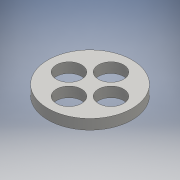
# Autodesk Inventor part: wheel
Saved by Autodesk Inventor 2016 (Build 200138000, 138)
## iProperties
Created: 2016-04-07
Part Number: wheel
Material: Generic
Document SubType Name: Modeling
Designer: hesaon
Density: 1 g/cm^3
Appearance: Default
Author: hesaon
Autodesk Inventor part; units mm, degrees
ref_plane "YZ Plane" through (0, 0, 0) normal (1, 0, 0) x (0, 1, 0)
ref_plane "XZ Plane" through (0, 0, 0) normal (0, 1, 0) x (-1, 0, 0)
ref_plane "XY Plane" through (0, 0, 0) normal (0, 0, 1) x (1, 0, 0)
sketch "Sketch1" plane through (0, 0, 0) normal (0, 0, 1) x (1, 0, 0)
  circle A0 centre (0, 0) radius 25
  arc A1 (-1.118, 1) -> (1.118, 1) centre (0, 0) ccw
  line L0 (0, 1) -> (1.118, 1)
  line L1 (1.118, 1) -> (0, 1)
  line L2 (0, 1) -> (-1.118, 1)
  dimension "d0" = 50
  dimension "d3" = 1
  dimension "d4" = 1.5
  dimension "d5" = 2.2361
  dimension "d6" = 1.118
  constraints: 6 end point, 2 centre point, 2 coincident, 2 point on circle, 1 collinear, 1 horizontal
  measures "d0" diameter of A0
  measures "d3" distance of L0.start point (0, 0)
  measures "d4" radius of A1
  measures "d5" distance of L0.end L2.end
  measures "d6" horizontal distance of point (0, 0) L2.end
extrude "Extrusion1" add sketch "Sketch1" along normal blind 4
sketch "Sketch2" plane through (0, 0, 4) normal (0, 0, 1) x (1, 0, 0)
  circle A0 centre (0, 0) radius 25 projected
  circle A1 centre (0, 0) radius 25
  constraints: 1 centre point, 1 coincident
extrude "Extrusion2" add sketch "Sketch2" along normal blind 2
sketch "Sketch3" plane through (0, 0, 0) normal (0, 0, -1) x (-1, 0, 0)
  point P0 (0, 0)
sketch "Sketch4" plane through (0, 0, 6) normal (0, 0, 1) x (1, 0, 0)
  circle A0 centre (12.5, 0) radius 7.5
  circle A1 centre (0, 12.5) radius 7.5
  circle A2 centre (-12.5, 0) radius 7.5
  circle A3 centre (0, -12.5) radius 7.5
  point P0 (0, 0)
  dimension "d14" = 15
  dimension "d15" = 12.5
  dimension "d18" = 360
  constraints: 4 centre point, 9 other
  measures "d14" diameter of A0
  measures "d15" distance of point (0, 0) A0.centre
extrude "Extrusion3" cut sketch "Sketch4" against normal through all
body "Solid1"
